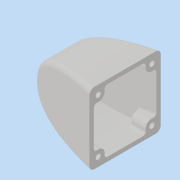
# Autodesk Inventor part: Fore
Saved by Autodesk Inventor 2017 (Build 210142000, 142)
## iProperties
Created: 2017-02-01
Part Number: Fore
Material: Generic
Document SubType Name: Modeling
Designer: techn
Density: 1 g/cm^3
Appearance: Default
Author: techn
Autodesk Inventor part; units mm, degrees
ref_plane "YZ Plane" through (0, 0, 0) normal (1, 0, 0) x (0, 1, 0)
ref_plane "XZ Plane" through (0, 0, 0) normal (0, 1, 0) x (-1, 0, 0)
ref_plane "XY Plane" through (0, 0, 0) normal (0, 0, 1) x (1, 0, 0)
sketch "Sketch1" plane through (0, 0, 0) normal (0, 0, 1) x (1, 0, 0)
  line L0 (0, 0) -> (0, 31.75)
  line L1 (0, 15.875) -> (-31.75, 15.875)
  line L2 (0, 31.75) -> (-31.75, 31.75) construction
  line L3 (-31.75, 31.75) -> (-31.75, 15.875) construction
  spline S0 degree 2 poles (0, 31.75) (-31.75, 31.75) (-31.75, 15.875) knots 1 1 1 2 2 2
  line L4 (0, 0) -> (-31.75, 0) construction
  line L5 (-31.75, 0) -> (-31.75, 15.875) construction
  spline S1 degree 2 poles (0, 0) (-31.75, 0) (-31.75, 15.875) knots 1 1 1 2 2 2
  dimension "d0" = 31.75
  dimension "d1" = 31.75
  constraints: 4 end point, 2 perpendicular, 1 horizontal, 1 midpoint, 1 symmetric about line, 1 vertical, 6 other
  measures "d0" distance of L0.start L0.end
  measures "d1" distance of L1.start L1.end
extrude "Extrusion1" add sketch "Sketch1" along normal blind 31.75
sketch "Sketch2" plane through (0, 0, 0) normal (0, 1, 0) x (-1, 0, 0)
  line L0 (31.75, 0) -> (31.75, 31.75) projected
  line L1 (31.75, 0) -> (31.75, 7.62)
  line L2 (0, 0) -> (0, 31.75) projected
  line L3 (31.75, 7.62) -> (0, 0)
  line L4 (0, 0) -> (31.75, 0)
  line L5 (31.75, 31.75) -> (31.75, 24.13)
  line L6 (31.75, 24.13) -> (0, 31.75)
  line L7 (0, 31.75) -> (31.75, 31.75)
  dimension "d4" = 7.62
  dimension "d5" = 7.62
  constraints: 12 end point, 2 perpendicular, 1 point on line
  measures "d4" distance of L0.start L1.end
  measures "d5" distance of L0.end L5.end
extrude "Extrusion2" cut sketch "Sketch2" along normal blind 31.75 contours L4 L3 L0 | L6 L7 L0
fillet "Fillet1" radius 2.286 4 edges at (-19.2983, 29.5323, 4.6316) (-19.2983, 2.2177, 4.6316) (-19.2983, 29.5323, 27.1184) (-19.2983, 2.2177, 27.1184)
shell "Shell1" thickness 1.905 removed faces 1 at (0, 21.1667, 11.367)
sketch "Sketch6" plane through (0, 2.286, 31.75) normal (1, 0, 0) x (0, 0, -1)
  line L0 (29.7909, 27.178) -> (29.7909, 0) projected
  line L1 (29.3991, -0.381) -> (2.3509, -0.381) projected
  line L2 (1.9591, 0) -> (1.9591, 27.178) projected
  line L3 (2.3509, 27.559) -> (29.3991, 27.559) projected
  line L4 (0, 0) -> (0, 27.178) projected
  line L5 (29.3991, -2.286) -> (2.3509, -2.286) projected
  line L6 (31.75, 0) -> (31.75, 27.178) projected
  line L7 (29.3991, 29.464) -> (2.3509, 29.464) projected
  line L8 (22.3277, 13.589) -> (9.4223, 13.589) projected
  circle A0 centre (3.937, 25.527) radius 1.143
  circle A1 centre (3.937, 25.527) radius 2.8575
  circle A2 centre (3.937, 1.651) radius 2.8575
  circle A3 centre (3.937, 1.651) radius 1.143
  circle A4 centre (27.813, 1.651) radius 2.8575
  circle A5 centre (27.813, 1.651) radius 1.143
  circle A6 centre (27.813, 25.527) radius 2.8575
  circle A7 centre (27.813, 25.527) radius 1.143
  point P0 (31.75, -2.286)
  point P1 (15.875, 13.589)
  dimension "d40" = 2.286
  dimension "d41" = 5.715
  dimension "d42" = 3.937
  dimension "d43" = 3.937
  dimension "d46" = 360
  constraints: 8 centre point, 4 coincident, 1 midpoint, 26 other
  measures "d40" diameter of A0
  measures "d41" diameter of A1
  measures "d42" distance from line of L4 A0.centre
  measures "d43" distance from line of A0.centre L7
extrude "Extrusion8" add sketch "Sketch6" against normal blind 6.35 contours A6 | A4 | A1 | A2
extrude "Extrusion9" cut sketch "Sketch6" against normal blind 6.985 contours A0 | A3 | A5 | A7
extrude "Extrusion10" cut sketch "Sketch2" along normal through all contours L4 L3 L0 | L6 L7 L0
fillet "Fillet3" radius 1.27 8 edges at (-3.177, 29.8024, 25.7618) (-2.934, 25.2551, 29.0867) (-3.1769, 1.9476, 5.9882) (-2.934, 6.4949, 2.6633) (-3.1769, 1.9476, 25.7618) (-2.934, 6.4949, 29.0867) (-2.934, 25.2551, 2.6633) (-3.177, 29.8024, 5.9882)
body "Solid1"
